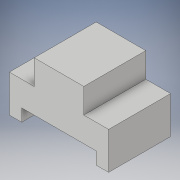
# Autodesk Inventor part: Part5
Saved by Autodesk Inventor 2017 (Build 210142000, 142)
## iProperties
Created: 2016-11-03
Part Number: Part5
Material: Generic
Document SubType Name: Modeling
Designer: s411888
Density: 1 g/cm^3
Appearance: Default
Author: s411888
Autodesk Inventor part; units mm, degrees
ref_plane "YZ Plane" through (0, 0, 0) normal (1, 0, 0) x (0, 1, 0)
ref_plane "XZ Plane" through (0, 0, 0) normal (0, 1, 0) x (-1, 0, 0)
ref_plane "XY Plane" through (0, 0, 0) normal (0, 0, 1) x (1, 0, 0)
sketch "Sketch1" plane through (0, 0, 0) normal (0, 0, 1) x (1, 0, 0)
  line L0 (-31.3679, 2.2573) -> (-25.0179, 2.2573)
  line L1 (-25.0179, 2.2573) -> (-25.0179, -16.7927)
  line L2 (-25.0179, -16.7927) -> (-31.3679, -16.7927)
  line L3 (-31.3679, -16.7927) -> (-31.3679, 2.2573)
  line L4 (-31.3679, 2.2573) -> (19.4321, 2.2573)
  line L5 (19.4321, 2.2573) -> (19.4321, -10.4427)
  line L6 (19.4321, -10.4427) -> (-31.3679, -10.4427)
  line L7 (-31.3679, -10.4427) -> (-31.3679, 2.2573)
  line L8 (19.4321, 2.2573) -> (13.0821, 2.2573)
  line L9 (13.0821, 2.2573) -> (13.0821, -16.7927)
  line L10 (13.0821, -16.7927) -> (19.4321, -16.7927)
  line L11 (19.4321, -16.7927) -> (19.4321, 2.2573)
  line L12 (-31.3679, 2.2573) -> (-18.6679, 2.2573)
  line L13 (-18.6679, 2.2573) -> (-18.6679, 14.9573)
  line L14 (-18.6679, 2.2573) -> (6.7321, 2.2573)
  line L15 (6.7321, 2.2573) -> (6.7321, 14.9573)
  line L16 (6.7321, 14.9573) -> (-18.6679, 14.9573)
  line L17 (-18.6679, 14.9573) -> (-18.6679, 2.2573)
  point P0 (0, 0)
  dimension "d0" = 6.35
  dimension "d1" = 19.05
  dimension "d2" = 50.8
  dimension "d3" = 12.7
  dimension "d4" = 6.35
  dimension "d5" = 19.05
  dimension "d7" = 12.7
  dimension "d8" = 25.4
  dimension "d9" = 12.7
  constraints: 36 end point, 8 parallel, 5 horizontal, 5 perpendicular
  measures "d0" distance of L1.end L2.end
  measures "d1" distance of L0.end L1.end
  measures "d2" distance of L5.end L6.end
  measures "d3" distance of L4.end L5.end
  measures "d4" distance of L10.end L9.end
  measures "d5" distance of L9.end L8.end
  measures "d7" distance of L13.end L12.end
  measures "d8" distance of L16.end L15.end
  measures "d9" distance of L15.end L14.end
extrude "Extrusion1" add sketch "Sketch1" along normal blind 31.75
body "Solid1"
